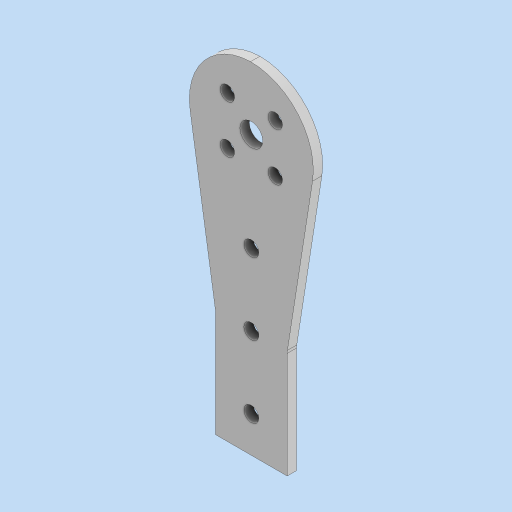
# Autodesk Inventor part: Arm Plate2
Saved by Autodesk Inventor 2024 (Build 280153000, 153)
## iProperties
Created: 2023-10-19
Part Number: Arm Plate2
Material: Generic
Document SubType Name: Modeling
Designer: ellen
Density: 1 g/cm^3
Appearance: Default
Author: ellen
Autodesk Inventor part; units mm, degrees
ref_plane "YZ Plane" through (0, 0, 0) normal (1, 0, 0) x (0, 1, 0)
ref_plane "XZ Plane" through (0, 0, 0) normal (0, 1, 0) x (-1, 0, 0)
ref_plane "XY Plane" through (0, 0, 0) normal (0, 0, 1) x (1, 0, 0)
sketch "Sketch1" plane through (0, 0, 0) normal (0, 0, 1) x (1, 0, 0)
  line L0 (44.45, 76.2) -> (0, 76.2)
  line L1 (0, 76.2) -> (0, 53.975)
  circle A0 centre (22.225, 53.975) radius 4.05
  circle A1 centre (22.225, 19.05) radius 2.6543
  circle A2 centre (22.225, -6.35) radius 2.6543
  line L2 (0, 53.975) -> (9.525, -6.35)
  line L3 (44.45, 53.975) -> (34.925, -6.35)
  line L4 (9.525, -6.35) -> (34.925, -6.35)
  line L5 (44.45, 53.975) -> (44.45, 76.2)
  circle A3 centre (22.225, -31.75) radius 2.6543
  line L6 (22.225, 76.2) -> (22.225, -33.1406) construction
  line L7 (34.925, -6.35) -> (34.925, -44.45)
  line L8 (34.925, -6.35) -> (73.025, -6.35) construction
  line L9 (34.925, -44.45) -> (9.525, -44.45)
  line L10 (9.525, -44.45) -> (9.525, -6.35)
  point P0 (0, 0)
  point P1 (24.8793, -6.35)
  point P2 (19.5707, -6.35)
  point P3 (22.225, -6.35)
  dimension "d0" = 44.45
  dimension "d2" = 8.1
  dimension "d3" = 5.3086
  dimension "d4" = 5.3086
  dimension "d5" = 22.225
  dimension "d8" = 22.225
  dimension "d9" = 22.225
  dimension "d44" = 5.3086
  dimension "d50" = 90
  dimension "d51" = 34.925
  dimension "d53" = 12.7
  dimension "d54" = 25.4
  dimension "d55" = 25.4
  dimension "d56" = 0
  constraints: 22 end point, 4 centre point, 4 perpendicular, 2 horizontal, 2 midpoint, 2 parallel, 2 vertical
  measures "d0" distance of L0.end L0.start
  measures "d2" diameter of A0
  measures "d3" diameter of A1
  measures "d4" diameter of A2
  measures "d5" distance of A0.centre L6.start
  measures "d8" distance from line of L5 A1.centre
  measures "d9" distance from line of L5 A2.centre
  measures "d44" diameter of A3
  measures "d50" angle of L7 L8
  measures "d51" distance of A1.centre A0.centre
  measures "d53" distance from line of L9 A3.centre
  measures "d54" distance of point (22.225, -6.35) A3.centre
  measures "d55" distance of point (22.225, -6.35) A1.centre
  measures "d56" distance of point (22.225, -6.35) A2.centre
extrude "Extrusion1" add sketch "Sketch1" along normal blind 3.302 contours L5 L3 L4 A2 L2 L1 L0 | L7 L9 L10 L4 A2
fillet "Fillet9" radius 12.7 1 edges at (44.45, 53.975, 1.651)
fillet "Fillet10" radius 12.7 1 edges at (0, 53.975, 1.651)
fillet "Fillet11" radius 22.225 1 edges at (44.45, 76.2, 1.651)
fillet "Fillet12" radius 22.225 1 edges at (0, 76.2, 1.651)
sketch "Sketch3" plane through (0, 0, 3.302) normal (0, 0, 1) x (1, 0, 0)
  circle A0 centre (22.225, 53.975) radius 4.05 projected
  circle A1 centre (22.225, 53.975) radius 16
  circle A2 centre (22.225, 53.975) radius 8
  circle A3 centre (22.225, 53.975) radius 12
  line L0 (22.225, 53.975) -> (44.4383, 53.975) construction
  line L1 (22.225, 53.975) -> (39.1956, 70.9456)
  line L2 (22.225, 53.975) -> (46.225, 53.975) construction
  point P0 (0, 0)
  point P1 (30.7103, 62.4603)
  dimension "d28" = 24
  dimension "d26" = 32
  dimension "d27" = 16
  dimension "d40" = 45
  constraints: 6 end point, 3 coincident, 2 centre point, 2 horizontal, 1 equal length, 1 midpoint, 3 other
  measures "d26" diameter of A1
  measures "d27" diameter of A2
  measures "d40" angle of L2 L1
hole "Hole1" at (30.7103, 62.4603, 3.302) direction (0, 0, -1) diameter 5.1054 depth 14.1986 tip angle 118 clearance for "Flat Head Machine Screw (82)" size "#10" standard "Ansi Unified Screw Threads"
pattern_circular "Circular Pattern2" count 4 over 360 about axis through (22.225, 53.975, 0) along (0, 0, 1) of "Hole1"
fillet "Fillet15" radius 6.35 2 edges at (9.525, -6.35, 1.651) (34.925, -6.35, 1.651)
body "Solid1"
